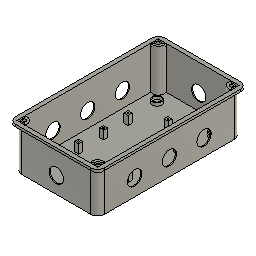
TP-electric-3310-217-0600 (Autodesk Fusion 360 design; units mm, degrees)
Autodesk Fusion 360 part; units mm, degrees
sketch "Main geometry" plane through (0, 0, 0) normal (0, 0, 1) x (1, 0, 0)
  line L0 (0, 0) -> (133, 0)
  line L1 (133, 0) -> (133, 224)
  line L2 (133, 224) -> (0, 224)
  line L3 (0, 224) -> (0, 0)
  line L4 (66.5, 224) -> (66.5, 0) construction
  line L5 (0, 112) -> (133, 112) construction
  line L6 (127, 218) -> (6, 218)
  line L7 (6, 218) -> (6, 6)
  line L8 (6, 6) -> (127, 6)
  line L9 (127, 6) -> (127, 218)
  line L10 (127, 218) -> (6, 6) construction
  line L11 (6, 218) -> (127, 6) construction
  line L12 (109, 198) -> (24, 198) construction
  line L13 (24, 198) -> (24, 26) construction
  line L14 (24, 26) -> (109, 26) construction
  line L15 (109, 26) -> (109, 198) construction
  line L16 (109, 198) -> (24, 26) construction
  line L17 (24, 198) -> (109, 26) construction
  circle A0 centre (24, 26) radius 7
  circle A1 centre (109, 26) radius 7
  circle A2 centre (24, 198) radius 7
  circle A3 centre (109, 198) radius 7
  line L18 (69.5, 175) -> (63.5, 175)
  line L19 (63.5, 175) -> (63.5, 169)
  line L20 (63.5, 169) -> (69.5, 169)
  line L21 (69.5, 169) -> (69.5, 175)
  line L22 (69.5, 175) -> (63.5, 169) construction
  line L23 (63.5, 175) -> (69.5, 169) construction
  line L24 (69.5, 49) -> (63.5, 49)
  line L25 (63.5, 49) -> (63.5, 55)
  line L26 (69.5, 55) -> (69.5, 49)
  line L27 (63.5, 55) -> (69.5, 55)
  line L28 (32.5, 72) -> (26.5, 72)
  line L29 (26.5, 72) -> (26.5, 78)
  line L30 (26.5, 78) -> (32.5, 78)
  line L31 (32.5, 78) -> (32.5, 72)
  line L32 (32.5, 72) -> (26.5, 78) construction
  line L33 (26.5, 72) -> (32.5, 78) construction
  line L34 (106.5, 78) -> (100.5, 78)
  line L35 (100.5, 78) -> (100.5, 72)
  line L36 (106.5, 72) -> (106.5, 78)
  line L37 (100.5, 72) -> (106.5, 72)
  line L38 (26.5, 146) -> (32.5, 146)
  line L39 (32.5, 146) -> (32.5, 152)
  line L40 (26.5, 152) -> (26.5, 146)
  line L41 (32.5, 152) -> (26.5, 152)
  line L42 (106.5, 146) -> (100.5, 146)
  line L43 (100.5, 146) -> (100.5, 152)
  line L44 (106.5, 152) -> (106.5, 146)
  line L45 (100.5, 152) -> (106.5, 152)
  line L46 (32.5, 115) -> (26.5, 115)
  line L47 (26.5, 115) -> (26.5, 109)
  line L48 (26.5, 109) -> (32.5, 109)
  line L49 (32.5, 109) -> (32.5, 115)
  line L50 (32.5, 115) -> (26.5, 109) construction
  line L51 (26.5, 115) -> (32.5, 109) construction
  line L52 (100.5, 115) -> (106.5, 115)
  line L53 (106.5, 115) -> (106.5, 109)
  line L54 (100.5, 109) -> (100.5, 115)
  line L55 (106.5, 109) -> (100.5, 109)
  circle A4 centre (29.5, 75) radius 1.25
  circle A5 centre (103.5, 75) radius 1.25
  circle A6 centre (103.5, 149) radius 1.25
  circle A7 centre (29.5, 149) radius 1.25
  circle A8 centre (29.5, 112) radius 1.25
  circle A9 centre (103.5, 112) radius 1.25
  circle A10 centre (66.5, 172) radius 1.25
  circle A11 centre (66.5, 52) radius 1.25
  line L56 (121.5, 212) -> (11.5, 212) construction
  line L57 (11.5, 212) -> (11.5, 12) construction
  line L58 (11.5, 12) -> (121.5, 12) construction
  line L59 (121.5, 12) -> (121.5, 212) construction
  line L60 (121.5, 212) -> (11.5, 12) construction
  line L61 (11.5, 212) -> (121.5, 12) construction
  circle A12 centre (11.5, 12) radius 4
  circle A13 centre (11.5, 12) radius 2.5
  circle A14 centre (121.5, 12) radius 2.5
  circle A15 centre (121.5, 12) radius 4
  circle A16 centre (11.5, 212) radius 2.5
  circle A17 centre (11.5, 212) radius 4
  circle A18 centre (121.5, 212) radius 2.5
  circle A19 centre (121.5, 212) radius 4
  line L62 (4.5, 4.5) -> (128.5, 4.5)
  line L63 (128.5, 4.5) -> (128.5, 219.5)
  line L64 (128.5, 219.5) -> (4.5, 219.5)
  line L65 (4.5, 219.5) -> (4.5, 4.5)
  circle A20 centre (24, 26) radius 5.5
  circle A21 centre (109, 26) radius 5.5
  circle A22 centre (24, 198) radius 5.5
  circle A23 centre (109, 198) radius 5.5
  line L66 (11.5, 12) -> (17.5, 6)
  line L67 (11.5, 12) -> (19.9853, 12) construction
  line L68 (11.5, 12) -> (6, 17.5)
  line L69 (121.5, 12) -> (127, 17.5)
  line L70 (121.5, 12) -> (115.5, 6)
  line L71 (121.5, 212) -> (115.5, 218)
  line L72 (121.5, 212) -> (127, 206.5)
  line L73 (11.5, 212) -> (17.5, 218)
  line L74 (11.5, 212) -> (6, 206.5)
  circle A24 centre (11.5, 12) radius 5.5
  circle A25 centre (121.5, 12) radius 5.5
  circle A26 centre (11.5, 212) radius 5.5
  circle A27 centre (121.5, 212) radius 5.5
  arc A28 (17.5, 6) -> (6, 17.5) centre (9.4655, 9.4655) ccw
  arc A29 (127, 17.5) -> (115.5, 6) centre (123.5345, 9.4655) ccw
  arc A30 (115.5, 218) -> (127, 206.5) centre (123.5345, 214.5345) ccw
  arc A31 (6, 206.5) -> (17.5, 218) centre (9.4655, 214.5345) ccw
  point P0 (66.5, 112)
  point P1 (66.5, 112)
  point P2 (66.5, 172)
  point P3 (29.5, 75)
  point P4 (29.5, 112)
  point P5 (66.5, 112)
  dimension "d1" = 133
  dimension "d10" = 224
  dimension "d11" = 121
  dimension "d12" = 212
  dimension "d13" = 85
  dimension "d14" = 172
  dimension "d15" = 14
  dimension "d18" = 85
  dimension "d19" = 172
  dimension "d21" = 6
  dimension "d22" = 6
  dimension "d23" = 60
  dimension "d24" = 6
  dimension "d25" = 6
  dimension "d26" = 37
  dimension "d27" = 37
  dimension "d28" = 6
  dimension "d29" = 6
  dimension "d30" = 37
  dimension "d31" = 2.5
  dimension "d32" = 2.5
  dimension "d33" = 2.5
  dimension "d40" = 110
  dimension "d41" = 200
  dimension "d42" = 8
  dimension "d43" = 5
  dimension "d46" = 110
  dimension "d47" = 200
  dimension "d68" = 45
  constraint horizontal L0
  constraint vertical L1
  constraint horizontal L2
  constraint vertical L3
  constraint coincident L0.start L3.end
  constraint midpoint L2 L4.start
  constraint midpoint L0 L4.end
  constraint midpoint L3 L5.start
  constraint midpoint L1 L5.end
  constraint perpendicular L6 L7
  constraint parallel L6 L8
  constraint parallel L7 L9
  constraint horizontal L6
  constraint coincident L10 P5
  constraint coincident L11 P5
  constraint midpoint L4 P5
  constraint perpendicular L12 L13
  constraint parallel L12 L14
  constraint parallel L13 L15
  constraint horizontal L12
  constraint coincident L16 P5
  constraint coincident L17 P5
  constraint coincident P5 P1
  constraint coincident L13.end L14.start
  constraint perpendicular L18 L19
  constraint parallel L18 L20
  constraint parallel L19 L21
  constraint horizontal L18
  constraint coincident L22 P2
  constraint coincident L23 P2
  constraint coincident L4 P2
  constraint symmetric L5 L18.start L24.start
  constraint symmetric L5 L18.end L24.end
  constraint symmetric L5 L19.end L25.end
  constraint symmetric L5 L20.end L26.start
  constraint perpendicular L28 L29
  constraint parallel L28 L30
  constraint parallel L29 L31
  constraint horizontal L28
  constraint coincident L32 P3
  constraint coincident L33 P3
  constraint symmetric L4 L28.start L35.end
  constraint symmetric L4 L28.end L36.start
  constraint symmetric L4 L29.end L34.start
  constraint symmetric L4 L30.end L34.end
  constraint symmetric L5 L28.start L39.end
  constraint symmetric L5 L28.end L40.start
  constraint symmetric L5 L29.end L38.start
  constraint symmetric L5 L30.end L38.end
  constraint symmetric L5 L34.start L42.start
  constraint symmetric L5 L34.end L42.end
  constraint symmetric L5 L35.end L43.end
  constraint symmetric L5 L36.start L44.start
  constraint perpendicular L46 L47
  constraint parallel L46 L48
  constraint parallel L47 L49
  constraint horizontal L46
  constraint coincident L50 P4
  constraint coincident L51 P4
  constraint coincident L5 P4
  constraint symmetric L4 L46.start L52.start
  constraint symmetric L4 L46.end L52.end
  constraint symmetric L4 L47.end L53.end
  constraint symmetric L4 L48.end L54.start
  constraint coincident P3 A4.centre
  constraint symmetric L4 A4 A5
  constraint symmetric L5 A4 A7
  constraint symmetric L5 A5 A6
  constraint coincident P4 A8.centre
  constraint symmetric L4 A8 A9
  constraint coincident P2 A10.centre
  constraint symmetric L5 A10 A11
  constraint perpendicular L56 L57
  constraint parallel L56 L58
  constraint parallel L57 L59
  constraint horizontal L56
  constraint coincident L60 P5
  constraint coincident L61 P5
  constraint coincident L57.end L58.start
  constraint concentric A12 A13
  constraint horizontal L67
  constraint coincident L8 L66.end
  constraint coincident L7 L68.end
  constraint parallel L66 L68
  constraint symmetric L4 L57.end L58.end
  constraint symmetric L4 L66.end L70.end
  constraint symmetric L4 L68.end L69.end
  constraint symmetric L5 L57.end L56.end
  constraint symmetric L5 L66.end L73.end
  constraint symmetric L5 L68.end L74.end
  constraint symmetric L5 L58.end L56.start
  constraint symmetric L5 L69.end L72.end
  constraint symmetric L5 L70.end L71.end
  constraint concentric A12 A24
  constraint tangent L7 A24
  constraint tangent A24 A28
  constraint symmetric L4 A28 A29
  constraint symmetric L5 A28 A31
  constraint symmetric L5 A29 A30
  measures "d1" distance of L0.start L0.end
  measures "d10" distance of L0.start L2.end
  measures "d11" distance of L7.end L8.end
  measures "d12" distance of L6 L8
  measures "d13" distance of L13.end L14.end L0.start
  measures "d14" distance of L12 L14
  measures "d15" diameter of A0
  measures "d21" distance of L19.end L20.end
  measures "d22" distance of L18.start L20.end
  measures "d23" distance of P5 P2
  measures "d24" distance of L28.end L29.end
  measures "d25" distance of L29.end L30.end
  measures "d26" distance of L5 P3
  measures "d27" distance of L4 P3
  measures "d28" distance of L47.end L48.end
  measures "d29" distance of L46.end L47.end
  measures "d30" distance of P5 P4
  measures "d31" diameter of A4
  measures "d32" diameter of A8
  measures "d33" diameter of A10
  measures "d40" distance of L57.end L58.end
  measures "d41" distance of L56 L58
  measures "d42" diameter of A12
  measures "d43" diameter of A13
  measures "d68" angle of L66 L67
extrude "Extrude1" add sketch "Main geometry" along normal blind 65 contours L62 L63 L64 L65 makes body 1
extrude "Extrude2" add sketch "Main geometry" along normal blind 1.5 contours L6 L9 L71 A27 | L6 L7 L8 L9 A28 A29 A30 A31 | L71 A27 A30 | A19 L71 L72 A27 | L9 L72 A27 | L6 L7 L73 A26 | L73 A26 A31 | A19 L71 L72 A27 | L72 A27 A30 | A17 L73 L74 A26 | A17 L73 L74 A26 | L74 A26 A31 | L9 L69 A25 | L69 A25 A29 | L7 L74 A26 | A15 L69 L70 A25 | L8 L9 L70 A25 | A15 L69 L70 A25 | L70 A25 A29 | L7 L68 A24 | L68 A24 A28 | L7 L8 L66 A24 | A12 L66 L68 A24 | A12 L66 L68 A24 | L66 A24 A28 bodies 1
extrude "Extrude3" add sketch "Main geometry" along normal blind 15 contours L18 L19 L20 L21 | L24 L25 L26 L27 | L28 L29 L30 L31 | L34 L35 L36 L37 | L38 L39 L40 L41 | L42 L43 L44 L45 | L46 L47 L48 L49 | L52 L53 L54 L55 bodies 1
extrude "Extrude4" add sketch "Main geometry" along normal blind 1.5 contours A4 | A5 | A6 | A7 | A8 | A9 | A10 | A11 bodies 1
extrude "Extrude5" add sketch "Main geometry" along normal blind 5.75 contours A0 | A1 | A2 | A3 bodies 1
extrude "Extrude6" add sketch "Main geometry" along normal blind 1.5 contours A20 | A21 | A22 | A23 bodies 1
extrude "Extrude7" add sketch "Main geometry" along normal blind 60.5 contours L6 L9 L71 A27 | A19 L71 L72 A27 | L9 L72 A27 | L6 L7 L73 A26 | A17 L73 L74 A26 | L9 L69 A25 | L7 L74 A26 | A15 L69 L70 A25 | L8 L9 L70 A25 | L7 L68 A24 | L7 L8 L66 A24 | A12 L66 L68 A24 picked at (124.291, 216.1333) picked at (6.5282, 212.4183) picked at (123.1573, 7.296) picked at (6.5282, 11.5817) bodies 1
extrude "Extrude8" add sketch "Main geometry" along normal blind 65 contours A18 A19 L71 L72 | A18 A19 L71 L72 | A16 A17 L73 L74 | A16 A17 L73 L74 | A14 A15 L69 L70 | A14 A15 L69 L70 | A12 A13 L66 L68 | A12 A13 L66 L68 bodies 1
extrude "Extrude9" add sketch "Main geometry" along normal blind 65 contours L71 A27 A30 | L73 A26 A31 | A19 L71 L72 A27 | L72 A27 A30 | A17 L73 L74 A26 | L74 A26 A31 | L69 A25 A29 | A15 L69 L70 A25 | L70 A25 A29 | L68 A24 A28 | A12 L66 L68 A24 | L66 A24 A28 picked at (118.7158, 207.8597) picked at (14.8407, 208.2962) picked at (118.7158, 16.1403) picked at (14.8407, 15.7038) bodies 1
ref_plane "WorkPlane1" through (0, 0, 65) normal (0, 0, 1) x (1, 0, 0)
sketch "Lip" plane through (0, 0, 65) normal (0, 0, 1) x (1, 0, 0)
  line L0 (0, 0) -> (133, 0)
  line L1 (133, 0) -> (133, 224)
  line L2 (133, 224) -> (0, 224)
  line L3 (0, 224) -> (0, 0)
  line L4 (128.5, 4.5) -> (128.5, 219.5)
  line L5 (128.5, 219.5) -> (4.5, 219.5)
  line L6 (4.5, 4.5) -> (128.5, 4.5)
  line L7 (4.5, 219.5) -> (4.5, 4.5)
extrude "Extrude10" add sketch "Lip" against normal blind 3.5 separate body makes body 2
combine "Combine1" operation add target body 2 tool bodies 1
chamfer "Chamfer1" distance 4.5 angle 35 4 edges at (128.5, 112, 61.5) (66.5, 4.5, 61.5) (4.5, 112, 61.5) (66.5, 219.5, 61.5) measured on face at (131.5, 147.8333, 61.5) measured on face at (131.5, 147.8333, 61.5) measured on face at (131.5, 147.8333, 61.5) measured on face at (131.5, 147.8333, 61.5) on bodies 2
fillet "Fillet1" radius 10 12 edges at (4.5, 4.5, 29.1745) (128.5, 4.5, 29.1745) (4.5, 219.5, 29.1745) (128.5, 219.5, 29.1745) (130.75, 221.75, 59.9245) (133, 224, 63.25) (2.25, 221.75, 59.9245) (0, 224, 63.25) (2.25, 2.25, 59.9245) (0, 0, 63.25) (130.75, 2.25, 59.9245) (133, 0, 63.25) on bodies 2
sketch "Sketch3" plane through (128.5, 0, 0) normal (1, 0, 0) x (0, 1, 0)
  line L0 (209.5, 0) -> (209.5, 58.3491)
  line L1 (209.5, 58.3491) -> (14.5, 58.3491)
  line L2 (14.5, 58.3491) -> (14.5, 0)
  line L3 (14.5, 0) -> (209.5, 0)
  line L4 (112, 0) -> (112, 58.3491) construction
  circle A0 centre (112, 24.75) radius 10.75
  line L5 (206.5, 1.5) -> (17.5, 1.5)
  circle A1 centre (60, 24.75) radius 10.75
  circle A2 centre (164, 24.75) radius 10.75
  dimension "d82" = 21.5
  dimension "d84" = 24.75
  dimension "d87" = 52
  dimension "d88" = 0
  constraint midpoint L3 L4.start
  constraint midpoint L1 L4.end
  constraint coincident L4 A0.centre
  measures "d82" diameter of A0
  measures "d84" distance of L3 A0.centre
sketch "Sketch4" plane through (0, 219.5, 0) normal (0, 1, 0) x (-1, 0, 0)
  line L0 (-118.5, 58.3491) -> (-118.5, 0)
  line L1 (-118.5, 0) -> (-14.5, 0)
  line L2 (-14.5, 0) -> (-14.5, 58.3491)
  line L3 (-14.5, 58.3491) -> (-118.5, 58.3491)
  line L4 (-66.5, 0) -> (-66.5, 58.3491) construction
  circle A0 centre (-66.5, 24.75) radius 10.75
  dimension "d89" = 21.5
  dimension "d90" = 24.75
  constraint midpoint L1 L4.start
  constraint midpoint L3 L4.end
  measures "d89" diameter of A0
  measures "d90" distance of L1 A0.centre
extrude "Extrude11" cut sketch "Sketch4" against normal up to surface (215 mm away) contours A0 bodies 2
extrude "Extrude12" cut sketch "Sketch3" against normal up to surface (124 mm away) contours A0 | A1 | A2 bodies 2
equation "d1 = outer_width"
equation "outer_width = 133 mm"
equation "inner_width = 121 mm"
equation "outer_height = 224 mm"
equation "inner_height = 212 mm"
equation "outer_depth = 91 mm"
equation "inner_depth = 85 mm"
equation "mounting_hole_width = 85 mm"
equation "mounting_hole_height = 172 mm"
equation "d10 = outer_height"
equation "d11 = inner_width"
equation "d12 = inner_height"
equation "d13 = mounting_hole_width"
equation "d14 = mounting_hole_height"
equation "d19 = mounting_hole_height"
equation "standoff_height = 120 mm"
equation "d23 = standoff_height / 2"
equation "d26 = standoff_square_side / 2"
equation "d27 = standoff_square_side / 2"
equation "d30 = standoff_square_side / 2"
equation "d31 = standoff_hole_diameter"
equation "d32 = standoff_hole_diameter"
equation "d33 = standoff_hole_diameter"
equation "standoff_square_side = 74 mm"
equation "standoff_hole_diameter = 2.5 mm"
equation "corner_hole_od = 8 mm"
equation "corner_hole_id = 5 mm"
equation "corner_hole_width = 110 mm"
equation "corner_hole_height = 200 mm"
equation "d40 = corner_hole_width"
equation "d41 = corner_hole_height"
equation "d42 = corner_hole_od"
equation "d43 = corner_hole_id"
equation "d46 = corner_hole_width"
equation "d47 = corner_hole_height"
equation "standoff_depth = 13.5 mm"
equation "lip_offset = 4.5 mm"
equation "d50 = -lip_offset"
equation "lip_height = 5.3 mm"
equation "lip_flat_height = 3.5 mm"
equation "bottom_box_outer_depth = 65 mm"
equation "d54 = bottom_box_outer_depth"
equation "wall_thickness = 1.5 mm"
equation "d57 = wall_thickness"
equation "d59 = standoff_depth + wall_thickness"
equation "d61 = wall_thickness"
equation "d63 = -wall_thickness"
equation "d64 = 4.25 mm + wall_thickness"
equation "d66 = wall_thickness"
equation "bottom_box_inner_depth = bottom_box_outer_depth - wall_thickness"
equation "d70 = bottom_box_inner_depth - 3 mm"
equation "d76 = bottom_box_outer_depth"
equation "d77 = -lip_flat_height"
equation "d79 = lip_offset"
equation "d84 = 14 mm + ( ( 21.5 / 2 ) * 1 mm )"
equation "d90 = ( ( 21.5 / 2 ) * 1 mm ) + 14 mm"
named bodies: "Lower body"
